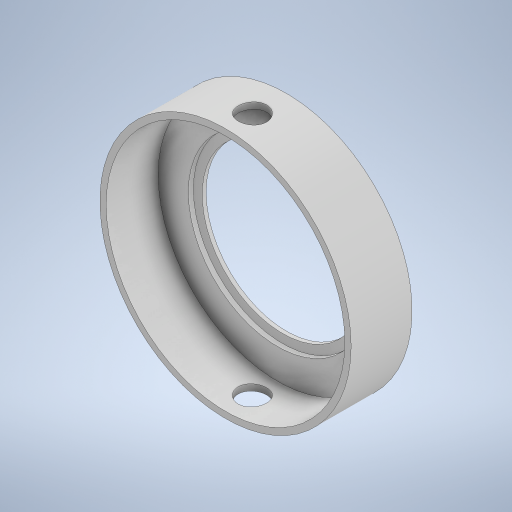
# Autodesk Inventor part: Diaphragm_lock
Saved by Autodesk Inventor 2023 (Build 270158000, 158)
## iProperties
Created: 2023-02-27
Part Number: Diaphragm_lock
Material: Generic
Document SubType Name: Modeling
Designer: maste
Density: 1 g/cm^3
Appearance: Default
Author: maste
Autodesk Inventor part; units mm, degrees
ref_plane "YZ Plane" through (0, 0, 0) normal (1, 0, 0) x (0, 1, 0)
ref_plane "XZ Plane" through (0, 0, 0) normal (0, 1, 0) x (-1, 0, 0)
ref_plane "XY Plane" through (0, 0, 0) normal (0, 0, 1) x (1, 0, 0)
sketch "Sketch1" plane through (0, 0, 0) normal (0, 0, 1) x (1, 0, 0)
  circle A0 centre (0, 0) radius 25
  dimension "d0" = 50
  constraints: 1 centre point, 1 coincident
  measures "d0" diameter of A0
extrude "Initial Cylinder" add sketch "Sketch1" along normal blind 4.78
sketch "Sketch2" plane through (0, 0, 4.78) normal (0, 0, 1) x (1, 0, 0)
  circle A0 centre (0, 0) radius 16
  dimension "d3" = 32
  constraints: 1 centre point, 1 coincident
  measures "d3" diameter of A0
extrude "Through-hole" cut sketch "Sketch2" against normal blind 548
sketch "Sketch3" plane through (0, 0, 4.78) normal (0, 0, 1) x (1, 0, 0)
  circle A0 centre (0, 0) radius 23.75
  dimension "d6" = 47.5
  constraints: 1 centre point, 1 coincident
  measures "d6" diameter of A0
extrude "snug ring fit" cut sketch "Sketch3" against normal blind 4
sketch "Sketch5" plane through (0, 0, 0) normal (0, 1, 0) x (-1, 0, 0)
  line L0 (25, 4.78) -> (-25, 4.78) projected
  line L1 (25, 0) -> (-25, 0) projected
  point P0 (0, 0)
  dimension "d16" = 4.78
  measures "d16" distance between parallel lines of L0 L1
sketch "Sketch6" plane through (0, 0, 0.78) normal (0, 0, 1) x (1, 0, 0)
  circle A0 centre (0, 0) radius 17.5
  dimension "d17" = 35
  constraints: 1 centre point, 1 coincident
  measures "d17" diameter of A0
extrude "Extrusion5" cut sketch "Sketch6" against normal blind 0.5
sketch "Sketch7" plane through (0, 0, 0) normal (0, 0, -1) x (-1, 0, 0)
  circle A0 centre (0, 0) radius 16 projected
  circle A1 centre (0, 0) radius 25 projected
extrude "Extrusion6" add sketch "Sketch7" along normal blind 1
sketch "Sketch8" plane through (0, 0, 0.28) normal (0, 0, 1) x (1, 0, 0)
  circle A0 centre (0, 0) radius 16 projected
  circle A1 centre (0, 0) radius 17.5 projected
  circle A2 centre (0, 0) radius 17.75
  dimension "d26" = 35.5
  constraints: 1 centre point, 1 coincident
  measures "d26" diameter of A2
extrude "Extrusion7" cut sketch "Sketch8" along normal mid plane 1 contours A1 | A2
sketch "Sketch9" plane through (0, 0, 4.78) normal (0, 0, 1) x (1, 0, 0)
  circle A0 centre (0, 0) radius 23.75 projected
  circle A1 centre (0, 0) radius 25 projected
extrude "Extrusion8" add sketch "Sketch9" along normal blind 0.35
sketch "Sketch10" plane through (0, 0, 5.13) normal (0, 0, 1) x (1, 0, 0)
  circle A0 centre (0, 0) radius 23.75 projected
  circle A1 centre (0, 0) radius 25 projected
  dimension "d30" = 1.25
  measures "d30" radial gap between concentric circles of A1 A0
extrude "Extrusion9" add sketch "Sketch10" along normal blind 6
sketch "Sketch4" plane through (0, 0, 0) normal (0, 1, 0) x (-1, 0, 0)
  line L0 (25, 4.78) -> (-25, 4.78) projected
  line L1 (0, 4.78) -> (0, 5.78)
  circle A0 centre (0, 5.78) radius 2.825
  point P0 (0, 0)
  dimension "d10" = 5.65
  dimension "d29" = 1
  constraints: 2 end point, 1 centre point, 1 coincident, 1 midpoint, 1 vertical
  measures "d10" diameter of A0
  measures "d29" distance of L1.start L1.end
extrude "Extrusion4" cut sketch "Sketch4" along normal mid plane 548
body "Solid1"
